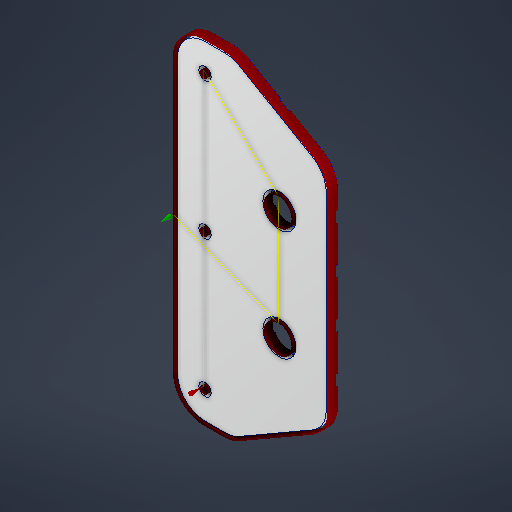
# Autodesk Inventor part: robocup_power_sw_plate
Saved by Autodesk Inventor 2026 (Build 300175000, 175)
## iProperties
Created: 2025-03-03
Part Number: robocup_power_sw_plate
Material: アルミニウム 6061
Document SubType Name: Sheet Metal
Designer: gisen
Density: 2.7 g/cm^3
Sheet Metal Rule: Default_mm
Appearance: アルミニウム - フラット
Sheet Metal Width: 0.000 mm
Sheet Metal Length: 0.000 mm
Sheet Metal Area: 0.000 mm^2
Author: gisen
Autodesk Inventor part; units mm, degrees
ref_plane "YZ Plane" through (0, 0, 0) normal (1, 0, 0) x (0, 1, 0)
ref_plane "XZ Plane" through (0, 0, 0) normal (0, 1, 0) x (-1, 0, 0)
ref_plane "XY Plane" through (0, 0, 0) normal (0, 0, 1) x (1, 0, 0)
sketch "スケッチ1" plane through (0, 0, 0) normal (0, 0, 1) x (1, 0, 0)
  line L0 (17, 0) -> (17, 80)
  line L1 (17, 80) -> (0, 80)
  line L2 (0, 80) -> (0, 0) construction
  line L3 (-17, 0) -> (-17, 80)
  line L4 (-17, 80) -> (0, 80)
  line L5 (-17, 0) -> (17, 0)
  dimension "d75" = 34
  dimension "d86" = 80
  constraints: 12 end point, 2 perpendicular, 2 symmetric about line, 1 coincident, 1 midpoint, 1 vertical
  measures "d75" distance between parallel lines of L0 L3
  measures "d86" distance of L0.start L0.end
extrude "プレート1" add sketch "スケッチ1" along normal blind 3
sketch "スケッチ3" plane through (0, 0, 3) normal (0, 0, 1) x (1, 0, 0)
  line L0 (-17, 80) -> (17, 80) construction
  line L1 (-17, 0) -> (-17, 80) construction
  line L2 (17, 80) -> (17, 0) construction
  line L3 (0, 0) -> (0, 80) construction
  line L4 (-17, 40) -> (17, 40) construction
  circle A0 centre (0, 60) radius 6
  circle A1 centre (0, 20) radius 6
  line L5 (17, 0) -> (-17, 0) projected
  point P0 (0, 0)
  dimension "d8" = 12
  dimension "d9" = 20
  dimension "d10" = 20
  constraints: 4 end point, 4 midpoint, 2 centre point, 2 point on line, 1 equal radius
  measures "d8" diameter of A0
  measures "d9" distance from line of L4 A0.centre
  measures "d10" distance from line of A1.centre L4
extrude "切り取り1" cut sketch "スケッチ3" against normal blind 3
sketch "スケッチ14" plane through (0, 0, 3) normal (0, 0, 1) x (1, 0, 0)
  line L0 (-17, 80) -> (17, 80)
  line L1 (-17, 0) -> (-17, 80)
  line L2 (17, 0) -> (-17, 0)
  line L3 (-37, 99.6299) -> (-37, -19.6299)
  line L4 (-37, -19.6299) -> (-17, -19.6299)
  line L5 (17, 0) -> (17, 80)
  line L6 (-17, -19.6299) -> (17, 0)
  line L7 (-37, 99.6299) -> (-17, 99.6299)
  line L8 (-17, 99.6299) -> (17, 80)
  line L9 (-27, 99.6299) -> (-27, -19.6299) construction
  line L10 (-27, 40) -> (-37, 40) construction
  circle A0 centre (-27, 89.6299) radius 2.25
  circle A1 centre (-27, -9.6299) radius 2.25
  circle A2 centre (-27, 40) radius 2.25
  point P0 (0, 0)
  dimension "d87" = 20
  dimension "d88" = 30
  dimension "d89" = 30
  dimension "d90" = 4.5
  dimension "d91" = 10
  dimension "d92" = 10
  measures "d87" distance of L3.start L7.end
  measures "d88" angle of L8 L0
  measures "d89" angle of L2 L6
  measures "d90" diameter of A0
  measures "d91" distance from line of A0.centre L7
  measures "d92" distance of L9.end A1.centre
sheet face with bend "面3" sketch "スケッチ14" thickness 3 toward (0, 0, -1) bend radius 0 contours L1 L2 L6 L4 L3 L7 L8 L0
bend "曲げ5"
fillet "フィレット4" radius 10 6 edges at (-37, 99.6299, 1.5) (-17, 99.6299, 1.5) (17, 80, 1.5) (17, 0, 1.5) (-17, -19.6299, 1.5) (-37, -19.6299, 1.5)
equation "\"d11\" = Thickness"
equation "\"d89\" = d88"
equation "\"d92\" = d91"
equation "\"d5\" = Thickness"
equation "\"d10\" = d9"
equation "\"d94\" = BendReliefWidth"
equation "\"d96\" = MinimumRemnant"
equation "\"d95\" = BendReliefDepth"
equation "\"BendReliefWidth\" = Thickness"
equation "\"BendReliefDepth\" = 0.5 * Thickness"
equation "\"CornerReliefSize\" = 4 * Thickness"
equation "\"MinimumRemnant\" = 2 * Thickness"
equation "\"GapSize\" = Thickness"
equation "\"Thickness\" = 3"
